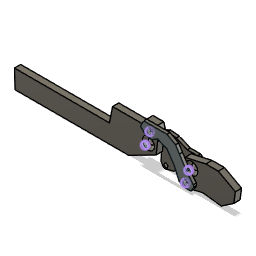
TestFingerJoint (Autodesk Fusion 360 design; units mm, degrees)
Autodesk Fusion 360 part; units mm, degrees
sketch "Sketch6" plane through (0, 0, 0) normal (0, 0, 1) x (1, 0, 0)
  line L0 (0, 0) -> (40, 0)
  line L1 (40, 0) -> (40, 20)
  line L2 (40, 20) -> (0, 20)
  line L3 (0, 20) -> (0, 0)
  line L4 (48, 20) -> (68, 20)
  line L5 (68, 20) -> (68, 0)
  line L6 (68, 0) -> (48, 0)
  line L7 (48, 0) -> (48, 20)
  line L8 (48, 13) -> (18, 13)
  line L9 (18, 13) -> (18, 7)
  line L10 (18, 7) -> (48, 7)
  line L11 (48, 7) -> (48, 13)
  line L12 (68, 13) -> (98, 13)
  line L13 (98, 13) -> (98, 7)
  line L14 (98, 7) -> (68, 7)
  line L15 (68, 7) -> (68, 13)
  line L16 (76, 0) -> (106, 0)
  line L17 (106, 0) -> (106, 20)
  line L18 (106, 20) -> (76, 20)
  line L19 (76, 20) -> (76, 0)
  dimension "d15" = 40
  dimension "d16" = 20
  dimension "d17" = 20
  dimension "d18" = 20
  dimension "d19" = 8
  dimension "d20" = 6
  dimension "d21" = 30
  dimension "d22" = 7
  dimension "d26" = 7
  dimension "d27" = 6
  dimension "d28" = 30
  dimension "d29" = 30
  dimension "d30" = 20
  dimension "d31" = 8
  constraint horizontal L0
  constraint vertical L1
  constraint horizontal L2
  constraint vertical L3
  constraint coincident L0.start L3.end
  constraint horizontal L4
  constraint vertical L5
  constraint horizontal L6
  constraint vertical L7
  constraint collinear L0 L6
  constraint horizontal L8
  constraint vertical L9
  constraint horizontal L10
  constraint vertical L11
  constraint coincident L7 L8.start
  constraint horizontal L12
  constraint vertical L13
  constraint horizontal L14
  constraint vertical L15
  constraint coincident L5 L12.start
  constraint horizontal L16
  constraint vertical L17
  constraint horizontal L18
  constraint vertical L19
  constraint collinear L0 L16
  measures "d15" distance of L0.start L0.end
  measures "d16" distance of L0.start L2.end
  measures "d17" distance of L5.end L6.end
  measures "d18" distance of L4.start L6.end
  measures "d19" distance of L1 L7
  measures "d20" distance of L8 L10
  measures "d21" distance of L8.start L8.end
  measures "d22" distance of L6 L10
  measures "d26" distance of L6 L14
  measures "d27" distance of L12.end L13.end
  measures "d28" distance of L12.start L12.end
  measures "d29" distance of L16.start L16.end
  measures "d30" distance of L16.start L18.end
  measures "d31" distance of L5 L19
extrude "Extrude6" add sketch "Sketch6" along normal blind 20 contours L0 L1 L2 L3 L8 L9 L10 | L1 L8 L9 L10 | L12 L13 L14 L19 | L12 L13 L14 L16 L17 L18 L19 makes body 1 at (13.3333, 0, 6.6667) makes body 2 at (96, 20, 6.6667)
extrude "Extrude7" add sketch "Sketch6" along normal blind 20 separate body contours L1 L8 L9 L10 | L1 L7 L8 L10 L11 | L4 L5 L6 L7 L11 L15 | L5 L12 L14 L15 L19 | L12 L13 L14 L19 makes body 3
sketch "Sketch7" plane through (0, 20, 0) normal (0, 1, 0) x (-1, 0, 0)
  line L0 (-68, 0) -> (-48, 0)
  line L1 (-48, 0) -> (-48, 20)
  line L2 (-48, 20) -> (-68, 20)
  line L3 (-68, 20) -> (-68, 0)
  line L4 (-98, 0) -> (-68, 0)
  line L5 (-68, 0) -> (-68, 20)
  line L6 (-68, 20) -> (-98, 20)
  line L7 (-98, 20) -> (-98, 0)
  line L8 (-48, 0) -> (-18, 0)
  line L9 (-18, 0) -> (-18, 20)
  line L10 (-18, 20) -> (-48, 20)
  line L11 (-48, 20) -> (-48, 0)
  line L12 (-98, 20) -> (-68, 20)
  line L13 (-68, 20) -> (-68, 15)
  line L14 (-68, 15) -> (-98, 15)
  line L15 (-98, 15) -> (-98, 20)
  line L16 (-98, 0) -> (-68, 0)
  line L17 (-68, 0) -> (-68, 5)
  line L18 (-68, 5) -> (-98, 5)
  line L19 (-98, 5) -> (-98, 0)
  line L20 (-48, 0) -> (-18, 0)
  line L21 (-18, 0) -> (-18, 5)
  line L22 (-18, 5) -> (-48, 5)
  line L23 (-48, 5) -> (-48, 0)
  line L24 (-18, 20) -> (-48, 20)
  line L25 (-48, 20) -> (-48, 15)
  line L26 (-48, 15) -> (-18, 15)
  line L27 (-18, 15) -> (-18, 20)
  dimension "d36" = 5
  dimension "d37" = 5
  dimension "d38" = 5
  dimension "d39" = 5
  constraint horizontal L12
  constraint vertical L13
  constraint horizontal L14
  constraint vertical L15
  constraint coincident L3 L13.end
  constraint coincident L6.end L7.start
  constraint horizontal L16
  constraint vertical L17
  constraint horizontal L18
  constraint vertical L19
  constraint coincident L5 L17.end
  constraint coincident L4.start L7.end
  constraint horizontal L20
  constraint vertical L21
  constraint horizontal L22
  constraint vertical L23
  constraint coincident L9 L21.end
  constraint coincident L0.end L1.start
  constraint horizontal L24
  constraint vertical L25
  constraint horizontal L26
  constraint vertical L27
  constraint coincident L11 L25.end
  constraint coincident L9.end L10.start
  measures "d36" distance of L6.end L14.end
  measures "d37" distance of L9.end L26.end
  measures "d38" distance of L4.start L18.end
  measures "d39" distance of L8.end L21.end
extrude "Extrude8" cut sketch "Sketch7" against normal blind 20 contours L3 L4 L5 L7 L16 L17 L18 L19 | L1 L8 L9 L11 L20 L21 L22 L23 | L3 L5 L6 L7 L12 L13 L14 L15 | L1 L9 L10 L11 L24 L25 L26 L27 bodies 3
sketch "Sketch8" plane through (0, 20, 0) normal (0, 1, 0) x (-1, 0, 0)
  line L0 (-40, 0) -> (0, 0)
  line L1 (0, 0) -> (0, 20)
  line L2 (0, 20) -> (-40, 20)
  line L3 (-40, 20) -> (-40, 0)
  line L4 (-103, 15.5) -> (-15, 15.5)
  line L5 (-15, 15.5) -> (-15, 4.5)
  line L6 (-15, 4.5) -> (-103, 4.5)
  line L7 (-103, 4.5) -> (-103, 15.5)
  line L8 (-98, 5) -> (-98, 15)
  line L9 (-68, 20) -> (-48, 20)
  point P0 (-18, 15)
  dimension "d43" = 5
  dimension "d44" = 3
  dimension "d45" = 11
  dimension "d46" = 4.5
  constraint horizontal L4
  constraint vertical L5
  constraint horizontal L6
  constraint vertical L7
  measures "d43" distance of L7 L8
  measures "d44" distance of L5 P0
  measures "d45" distance of L4.start L6.end
  measures "d46" distance of L4 L9
extrude "Extrude9" cut sketch "Sketch8" against normal blind 20 contours L3 L4 L6 L7 | L3 L4 L5 L6 bodies 1 2
sketch "Sketch9" plane through (0, 0, 20) normal (0, 0, 1) x (1, 0, 0)
  line L0 (0, 20) -> (0, 0)
  line L1 (0, 0) -> (40, 0)
  line L2 (40, 0) -> (40, 20)
  line L3 (40, 20) -> (0, 20)
  line L4 (98, 13) -> (68, 13)
  line L5 (68, 13) -> (68, 7)
  line L6 (68, 7) -> (98, 7)
  line L7 (98, 7) -> (98, 13)
  line L8 (48, 13) -> (18, 13)
  line L9 (18, 13) -> (18, 7)
  line L10 (18, 7) -> (48, 7)
  line L11 (48, 7) -> (48, 13)
  circle A0 centre (21.5, 10) radius 2
  circle A1 centre (94.5, 10) radius 2
  dimension "d49" = 4
  dimension "d50" = 4
  dimension "d51" = 3.5
  dimension "d52" = 3.5
  dimension "d53" = 3
  dimension "d54" = 3
  measures "d49" diameter of A0
  measures "d50" diameter of A1
  measures "d51" distance of L9 A0.centre
  measures "d52" distance of L7 A1.centre
  measures "d53" distance of L4 A1.centre
  measures "d54" distance of L10 A0.centre
extrude "Extrude10" cut sketch "Sketch9" against normal blind 20 contours A0 | A1 bodies 1 2 3
fillet "Fillet1" radius 8 8 edges at (40, 20, 2.25) (40, 20, 17.75) (40, 0, 17.75) (40, 0, 2.25) (76, 20, 17.75) (76, 20, 2.25) (76, 0, 17.75) (76, 0, 2.25) on bodies 1 2
fillet "Fillet2" radius 5 4 edges at (48, 0, 10) (68, 0, 10) (68, 20, 10) (48, 20, 10) on bodies 3
fillet "Fillet3" radius 4 4 edges at (48, 10, 15) (68, 10, 15) (68, 10, 5) (48, 10, 5) on bodies 3
sketch "Sketch10" plane through (0, 0, 20) normal (0, 0, 1) x (1, 0, 0)
  arc A0 (32, 0) -> (40, 8) centre (32, 8) ccw
  line L0 (40, 8) -> (40, 12)
  arc A1 (40, 12) -> (32, 20) centre (32, 12) ccw
  line L1 (32, 20) -> (0, 20)
  line L2 (0, 20) -> (0, 0)
  line L3 (0, 0) -> (32, 0)
  circle A2 centre (21.5, 10) radius 2
  line L4 (22.4525, 22.3546) -> (97.1627, 3.9644)
  line L5 (97.1627, 3.9644) -> (95.5692, -2.509)
  line L6 (95.5692, -2.509) -> (20.859, 15.8812)
  line L7 (20.859, 15.8812) -> (22.4525, 22.3546)
  line L8 (84, 0) -> (106, 0)
  circle A3 centre (94.5, 10) radius 2
  circle A4 centre (25.5, 18) radius 2
  circle A5 centre (90.5, 2) radius 2
  circle A6 centre (94.5, 10) radius 2
  dimension "d63" = 6.6667
  dimension "d66" = 4
  dimension "d67" = 4
  dimension "d96" = 8
  dimension "d98" = 8
  dimension "d99" = 4
  dimension "d100" = 6
  dimension "d101" = 3.5
  dimension "d103" = 4
  dimension "d104" = 3.5
  dimension "d105" = 4
  constraint perpendicular L4 L5
  constraint perpendicular L6 L7
  constraint perpendicular L5 L6
  measures "d63" distance of L4 L6
  measures "d66" diameter of A4
  measures "d67" diameter of A5
  measures "d96" vertical distance of A3.centre A5.centre
  measures "d98" vertical distance of A2.centre A4.centre
  measures "d99" distance of L7 A4.centre
  measures "d100" distance of L5 A5.centre
  measures "d101" distance of L4 A5.centre
  measures "d103" horizontal distance of A2.centre A4.centre
  measures "d104" distance of L4 A4.centre
  measures "d105" horizontal distance of A5.centre A3.centre
extrude "Extrude11" add sketch "Sketch10" along normal blind 3 separate body contours L0 A1 L1 L4 L6 L7 | L0 A1 L4 L5 L6 L8 | L5 L6 L8 | A1 L1 L4 L7 makes body 4
extrude "Extrude12" cut sketch "Sketch10" against normal blind 20 contours A4 | A5 bodies 1 2
chamfer "Chamfer1" distance 2 angle 45 2 edges at (19.6353, 10.7232, 20) (92.6353, 10.7232, 20) on bodies 1 2
fillet "Fillet4" radius 3 4 edges at (18, 13, 10) (98, 13, 10) (18, 7, 10) (98, 7, 10) on bodies 3
fillet "Fillet5" radius 2 4 edges at (20.859, 15.8812, 21.5) (22.4525, 22.3546, 21.5) (97.1627, 3.9644, 21.5) (95.5692, -2.509, 21.5) on bodies 4
copy_body "Body->Comp1" bodies 1 removing the originals makes body 5 in component "Component"
copy_body "Body->Comp2" bodies 2 removing the originals makes body 6 in component "Component'"
copy_body "Body->Comp3" bodies 3 removing the originals makes body 7 in component "Component''"
copy_body "Body->Comp4" bodies 4 removing the originals makes body 8 in component "Component'''"
sketch "Sketch11" plane through (0, 0, 0) normal (0, 0, 1) x (1, 0, 0)
  line L0 (7, 19) -> (7, -3)
  line L1 (7, -3) -> (17.4217, -3)
  line L2 (17.4217, -3) -> (35, 6)
  line L3 (35, 6) -> (36, 14)
  line L4 (27, 19) -> (7, 19)
  line L5 (67, 17) -> (53.6443, 14)
  line L6 (53.6443, 14) -> (50.5462, 8.5837)
  line L7 (50.5462, 8.5837) -> (52, -1)
  line L8 (65, 0) -> (76.9497, -1.4937)
  line L9 (76.9497, -1.4937) -> (85, 4)
  line L10 (85, 4) -> (86, 11)
  line L11 (86, 11) -> (75, 17)
  line L12 (75, 17) -> (67, 17)
  line L13 (27, 19) -> (29, 23)
  line L14 (29, 23) -> (36, 23)
  line L15 (36, 23) -> (37, 19)
  line L16 (37, 19) -> (36, 14)
  line L17 (52, -1) -> (58.4026, -1.6282)
  line L18 (58.4026, -1.6282) -> (65, 0)
  constraint vertical L0
  constraint perpendicular L0 L1
  constraint perpendicular L3 L8
  constraint horizontal L12
  constraint horizontal L4
  constraint parallel L4 L14
extrude "Extrude13" add sketch "Sketch11" along normal blind 2 separate body makes body 9 at (17.1406, 11.6667, 0) makes body 10 at (61.8814, 10.3333, 0)
sketch "Sketch12" plane through (0, 0, 2) normal (0, 0, 1) x (1, 0, 0)
  line L0 (27, 19) -> (7, 19)
  line L1 (7, 19) -> (7, -3)
  line L2 (7, -3) -> (17.4217, -3)
  line L3 (17.4217, -3) -> (35, 6)
  line L4 (35, 6) -> (36, 14)
  line L5 (36, 14) -> (37, 19)
  line L6 (37, 19) -> (36, 23)
  line L7 (36, 23) -> (29, 23)
  line L8 (29, 23) -> (27, 19)
  line L9 (29, 23) -> (27, 19)
  line L10 (27, 19) -> (30, 16)
  line L11 (30, 16) -> (34, 15)
  line L12 (34, 15) -> (38.0159, 17.5)
  line L13 (38.0159, 17.5) -> (40.2914, 16.25)
  line L14 (40.2914, 16.25) -> (44, 15)
  line L15 (44, 15) -> (46, 12)
  line L16 (46, 12) -> (48.6074, 8.089)
  line L17 (48.6074, 8.089) -> (50.6634, 3.4975)
  line L18 (50.6634, 3.4975) -> (51.8645, 0.8152)
  line L19 (51.8645, 0.8152) -> (55.0151, -0.9155)
  line L20 (55.0151, -0.9155) -> (59.4478, -0.9155)
  line L21 (59.4478, -0.9155) -> (61.1353, 2.1564)
  line L22 (61.1353, 2.1564) -> (60.2916, 7.1489)
  line L23 (60.2916, 7.1489) -> (57.2315, 12.0174)
  line L24 (57.2315, 12.0174) -> (52, 16)
  line L25 (52, 16) -> (49.5037, 19.9716)
  line L26 (49.5037, 19.9716) -> (44, 23)
  line L27 (44, 23) -> (38, 23)
  line L28 (38, 23) -> (29, 23)
  constraint coincident L7.end L8.start
  constraint coincident L0.start L8.end
  constraint parallel L15 L16
  constraint parallel L17 L18
  constraint parallel L13 L19
  constraint horizontal L20
  constraint perpendicular L19 L21
  constraint parallel L23 L25
  constraint horizontal L27
  constraint parallel L7 L28
extrude "Extrude14" add sketch "Sketch12" along normal blind 2 separate body contours L5 L6 L7 L8 L9 L10 L11 L12 L28 | L5 L6 L12 L13 L14 L15 L16 L17 L18 L19 L20 L21 L22 L23 L24 L25 L26 L27 L28 makes body 11
sketch "Sketch13" plane through (0, 0, 4) normal (0, 0, 1) x (1, 0, 0)
  line L0 (44, 23) -> (29, 23)
  line L1 (29, 23) -> (27, 19)
  line L2 (27, 19) -> (30, 16)
  line L3 (30, 16) -> (34, 15)
  line L4 (34, 15) -> (38.0159, 17.5)
  line L5 (38.0159, 17.5) -> (40.2914, 16.25)
  line L6 (40.2914, 16.25) -> (44, 15)
  line L7 (44, 15) -> (48.6074, 8.089)
  line L8 (48.6074, 8.089) -> (51.8645, 0.8152)
  line L9 (51.8645, 0.8152) -> (55.0151, -0.9155)
  line L10 (55.0151, -0.9155) -> (59.4478, -0.9155)
  line L11 (59.4478, -0.9155) -> (61.1353, 2.1564)
  line L12 (61.1353, 2.1564) -> (60.2916, 7.1489)
  line L13 (60.2916, 7.1489) -> (57.2315, 12.0174)
  line L14 (57.2315, 12.0174) -> (52, 16)
  line L15 (52, 16) -> (49.5037, 19.9716)
  line L16 (49.5037, 19.9716) -> (44, 23)
  line L17 (29, 14) -> (25, 12)
  line L18 (25, 12) -> (24.3664, 7.5642)
  line L19 (24.3664, 7.5642) -> (28, 6)
  line L20 (28, 6) -> (34, 6)
  line L21 (34, 6) -> (35, 4)
  line L22 (35, 4) -> (39, 0)
  line L23 (39, 0) -> (45, -3)
  line L24 (45, -3) -> (49, -1)
  line L25 (49, -1) -> (51.995, 4.4521)
  line L26 (51.995, 4.4521) -> (56.2929, 6.3766)
  line L27 (56.2929, 6.3766) -> (58.9406, 7.5623)
  line L28 (58.9406, 7.5623) -> (62.1557, 9.5831)
  line L29 (62.1557, 9.5831) -> (60.9516, 12.272)
  line L30 (60.9516, 12.272) -> (57.6168, 14.914)
  line L31 (57.6168, 14.914) -> (51, 14.914)
  line L32 (51, 14.914) -> (44, 18)
  line L33 (44, 18) -> (38.3016, 18.5595)
  line L34 (38.3016, 18.5595) -> (33.6565, 16.457)
  line L35 (33.6565, 16.457) -> (30.1314, 14.8614)
  line L36 (30.1314, 14.8614) -> (29, 14)
  constraint horizontal L20
  constraint perpendicular L17 L21
  constraint parallel L17 L24
  constraint perpendicular L9 L25
  constraint perpendicular L8 L26
  constraint perpendicular L8 L27
  constraint perpendicular L13 L28
  constraint perpendicular L27 L29
  constraint horizontal L31
  constraint parallel L34 L35
extrude "Extrude15" add sketch "Sketch13" along normal blind 2 separate body contours L13 L14 L28 L29 L30 L31 | L3 L4 L5 L6 L7 L8 L13 L14 L25 L26 L27 L28 L31 L32 L33 L34 L35 | L3 L4 L5 L6 L7 L8 L17 L18 L19 L20 L21 L22 L23 L24 L25 L35 L36 makes body 12
extrude "Extrude16" add 2 faces at (61.8814, 10.3333, 0) (17.1406, 11.6667, 0) along direction (0, 0, -1) blind 2 on bodies 9 10 bodies 10 9 11 12
sketch "Sketch14" plane through (0, 0, 6) normal (0, 0, 1) x (1, 0, 0)
  line L0 (30.1314, 14.8614) -> (29, 14)
  line L1 (29, 14) -> (25, 12)
  line L2 (25, 12) -> (24.3664, 7.5642)
  line L3 (24.3664, 7.5642) -> (28, 6)
  line L4 (28, 6) -> (34, 6)
  line L5 (34, 6) -> (35, 4)
  line L6 (35, 4) -> (39, 0)
  line L7 (39, 0) -> (45, -3)
  line L8 (45, -3) -> (49, -1)
  line L9 (49, -1) -> (51.995, 4.4521)
  line L10 (51.995, 4.4521) -> (58.9406, 7.5623)
  line L11 (58.9406, 7.5623) -> (62.1557, 9.5831)
  line L12 (62.1557, 9.5831) -> (60.9516, 12.272)
  line L13 (60.9516, 12.272) -> (57.6168, 14.914)
  line L14 (57.6168, 14.914) -> (51, 14.914)
  line L15 (51, 14.914) -> (44, 18)
  line L16 (44, 18) -> (38.3016, 18.5595)
  line L17 (38.3016, 18.5595) -> (30.1314, 14.8614)
  circle A0 centre (58, 10) radius 1.85
  circle A1 centre (56, 2) radius 1.85
  circle A2 centre (30, 10) radius 1.85
  circle A3 centre (33, 19) radius 1.85
  dimension "d114" = 3.7
  dimension "d115" = 3.7
  dimension "d116" = 3.7
  dimension "d117" = 3.7
  measures "d114" diameter of A0
  measures "d115" diameter of A1
  measures "d116" diameter of A2
  measures "d117" diameter of A3
extrude "Extrude17" cut sketch "Sketch14" against normal blind 8 contours A0 | A1 | A2 | A3 bodies 9 10 11 12
chamfer "Chamfer2" distance 2 angle 45 2 edges at (28.2752, 10.669, 2) (56.2752, 10.669, 2) on bodies 9 10
move_body "Move1" bodies 12 to x (1, 0, 0) y (0, 1, 0) z (0, 0, 1) at (0, 0, -8)
sketch "Sketch15" plane through (0, 0, 4) normal (0, 0, 1) x (1, 0, 0)
  arc A0 (57.3996, 11.7499) -> (59.3165, 8.7002) centre (58, 10) ccw
  line L0 (57.3996, 11.7499) -> (57.2315, 12.0174)
  line L1 (57.2315, 12.0174) -> (52, 16)
  line L2 (52, 16) -> (49.5037, 19.9716)
  line L3 (49.5037, 19.9716) -> (44, 23)
  line L4 (44, 23) -> (29, 23)
  line L5 (29, 23) -> (27, 19)
  line L6 (27, 19) -> (30, 16)
  line L7 (30, 16) -> (34, 15)
  line L8 (34, 15) -> (38.0159, 17.5)
  line L9 (38.0159, 17.5) -> (40.2914, 16.25)
  line L10 (40.2914, 16.25) -> (44, 15)
  line L11 (44, 15) -> (48.6074, 8.089)
  line L12 (48.6074, 8.089) -> (51.8645, 0.8152)
  line L13 (51.8645, 0.8152) -> (55.0151, -0.9155)
  line L14 (55.0151, -0.9155) -> (59.4478, -0.9155)
  line L15 (59.4478, -0.9155) -> (61.1353, 2.1564)
  line L16 (61.1353, 2.1564) -> (60.2916, 7.1489)
  line L17 (60.2916, 7.1489) -> (59.3165, 8.7002)
  circle A1 centre (56, 2) radius 1.85
  circle A2 centre (33, 19) radius 1.85
  line L18 (56.4337, 9.0155) -> (60.9319, 3.36)
  line L19 (56.6883, 8.6954) -> (52, 16)
  constraint midpoint A0 L18.start
  constraint coincident L16 L18.end
  constraint coincident A0 L19.start
  constraint coincident L18 L19.start
  constraint coincident L1.end L2.start
extrude "Extrude18" cut sketch "Sketch15" against normal blind 2 contours A0 L16 L17 L18 | A0 L0 L1 L19 bodies 11
chamfer "Chamfer3" distance 2 angle 45 2 edges at (31.2752, 18.331, -2) (54.2752, 1.331, -2) on bodies 9 10
sketch "Sketch16" plane through (0, 0, 2) normal (0, 0, 1) x (1, 0, 0)
  line L0 (27, 19) -> (7, 19)
  line L1 (7, 19) -> (7, -3)
  line L2 (7, -3) -> (17.4217, -3)
  line L3 (17.4217, -3) -> (35, 6)
  line L4 (35, 6) -> (36, 14)
  line L5 (36, 14) -> (37, 19)
  line L6 (37, 19) -> (36, 23)
  line L7 (36, 23) -> (29, 23)
  line L8 (29, 23) -> (27, 19)
  circle A0 centre (33, 19) radius 1.85
  circle A1 centre (30, 10) radius 3.85
  line L9 (7, -3) -> (-55.6859, -3)
  line L10 (-55.6859, -3) -> (-57.0823, 34.1911)
  line L11 (-57.0823, 34.1911) -> (0.0915, 30.8262)
  line L12 (0.0915, 30.8262) -> (7, 19)
  constraint coincident L1.end L2.start
  constraint perpendicular L1 L9
  constraint coincident L0.end L1.start
extrude "Extrude19" add sketch "Sketch16" against normal blind 4 contours L1 L9 L10 L11 L12 bodies 9
sketch "Sketch17" plane through (0, 0, 2) normal (0, 0, 1) x (1, 0, 0)
  line L0 (27, 19) -> (7, 19)
  line L1 (7, 19) -> (0.0915, 30.8262)
  line L2 (0.0915, 30.8262) -> (-57.0823, 34.1911)
  line L3 (-57.0823, 34.1911) -> (-55.6859, -3)
  line L4 (-55.6859, -3) -> (17.4217, -3)
  line L5 (17.4217, -3) -> (35, 6)
  line L6 (35, 6) -> (36, 14)
  line L7 (36, 14) -> (37, 19)
  line L8 (37, 19) -> (36, 23)
  line L9 (36, 23) -> (29, 23)
  line L10 (29, 23) -> (27, 19)
  circle A0 centre (33, 19) radius 1.85
  circle A1 centre (30, 10) radius 3.85
  line L11 (-56.1315, 8.8703) -> (5, 8.8703)
  line L12 (5, 8.8703) -> (7, 19)
  constraint coincident L3 L11.start
  constraint horizontal L11
  constraint coincident L0.end L1.start
extrude "Extrude20" cut sketch "Sketch17" against normal blind 4 contours L1 L2 L3 L11 L12 bodies 9
sketch "Sketch18" plane through (0, 0, 2) normal (0, 0, 1) x (1, 0, 0)
  circle A0 centre (30, 10) radius 3.85
  circle A1 centre (33, 19) radius 1.85
  line L0 (7, 19) -> (5, 8.8703)
  line L1 (5, 8.8703) -> (-56.1315, 8.8703)
  line L2 (-56.1315, 8.8703) -> (-55.6859, -3)
  line L3 (-55.6859, -3) -> (17.4217, -3)
  line L4 (17.4217, -3) -> (35, 6)
  line L5 (35, 6) -> (36, 14)
  line L6 (36, 14) -> (37, 19)
  line L7 (37, 19) -> (36, 23)
  line L8 (36, 23) -> (29, 23)
  line L9 (29, 23) -> (27, 19)
  line L10 (27, 19) -> (7, 19)
  line L11 (-56.1315, 8.8703) -> (-6.3246, 8.8703)
  line L12 (-6.3246, 8.8703) -> (-6.3246, 2.9351)
  line L13 (-6.3246, 2.9351) -> (-56.1315, 2.9351)
  line L14 (-56.1315, 2.9351) -> (-56.1315, 8.8703)
  constraint horizontal L11
  constraint vertical L12
  constraint horizontal L13
  constraint vertical L14
  constraint coincident L1.end L2.start
extrude "Extrude21" add sketch "Sketch18" along normal blind 4 contours L1 L2 L11 L12 L13 bodies 9
extrude "Extrude22" add 1 faces at (-39.4549, 6.8919, 6) along direction (0, 0, 1) blind 4 on bodies 9 bodies 9
sketch "Sketch19" plane through (0, 0, -4) normal (0, 0, -1) x (-1, 0, 0)
  circle A0 centre (-30, 10) radius 1.85
  circle A1 centre (-58, 10) radius 1.85
  line L0 (-29, 14) -> (-30.1314, 14.8614)
  line L1 (-30.1314, 14.8614) -> (-38.3016, 18.5595)
  line L2 (-38.3016, 18.5595) -> (-44, 18)
  line L3 (-44, 18) -> (-51, 14.914)
  line L4 (-51, 14.914) -> (-57.6168, 14.914)
  line L5 (-57.6168, 14.914) -> (-60.9516, 12.272)
  line L6 (-60.9516, 12.272) -> (-62.1557, 9.5831)
  line L7 (-62.1557, 9.5831) -> (-58.9406, 7.5623)
  line L8 (-58.9406, 7.5623) -> (-51.995, 4.4521)
  line L9 (-51.995, 4.4521) -> (-49, -1)
  line L10 (-49, -1) -> (-45, -3)
  line L11 (-45, -3) -> (-39, 0)
  line L12 (-39, 0) -> (-35, 4)
  line L13 (-35, 4) -> (-34, 6)
  line L14 (-34, 6) -> (-28, 6)
  line L15 (-28, 6) -> (-24.3664, 7.5642)
  line L16 (-24.3664, 7.5642) -> (-25, 12)
  line L17 (-25, 12) -> (-29, 14)
  line L18 (-51.995, 4.4521) -> (-42, -1.5)
  constraint coincident L8.end L9.start
  constraint midpoint L11 L18.end
extrude "Extrude23" cut sketch "Sketch19" against normal blind 2 contours L9 L10 L11 L18 bodies 12
sketch "Sketch20" plane through (0, 0, -4) normal (0, 0, -1) x (-1, 0, 0)
  line L0 (-51.995, 4.4521) -> (-42, -1.5)
  line L1 (-42, -1.5) -> (-39, 0)
  line L2 (-39, 0) -> (-35, 4)
  line L3 (-35, 4) -> (-34, 6)
  line L4 (-34, 6) -> (-28, 6)
  line L5 (-28, 6) -> (-24.3664, 7.5642)
  line L6 (-24.3664, 7.5642) -> (-25, 12)
  line L7 (-25, 12) -> (-29, 14)
  line L8 (-29, 14) -> (-30.1314, 14.8614)
  line L9 (-30.1314, 14.8614) -> (-38.3016, 18.5595)
  line L10 (-38.3016, 18.5595) -> (-44, 18)
  line L11 (-44, 18) -> (-51, 14.914)
  line L12 (-51, 14.914) -> (-57.6168, 14.914)
  line L13 (-57.6168, 14.914) -> (-60.9516, 12.272)
  line L14 (-60.9516, 12.272) -> (-62.1557, 9.5831)
  line L15 (-62.1557, 9.5831) -> (-58.9406, 7.5623)
  line L16 (-58.9406, 7.5623) -> (-51.995, 4.4521)
  circle A0 centre (-30, 10) radius 1.85
  circle A1 centre (-58, 10) radius 1.85
  line L17 (-42, -1.5) -> (-36, -3)
  line L18 (-36, -3) -> (-34.141, 0.1217)
  line L19 (-34.141, 0.1217) -> (-34.5, 5)
  constraint coincident L0.end L1.start
  constraint perpendicular L0 L18
  constraint midpoint L3 L19.end
extrude "Extrude24" add sketch "Sketch20" against normal blind 2 contours L1 L2 L3 L17 L18 L19 bodies 12
sketch "Sketch21" plane through (0, 0, -4) normal (0, 0, -1) x (-1, 0, 0)
  line L0 (-51.995, 4.4521) -> (-42, -1.5)
  line L1 (-42, -1.5) -> (-36, -3)
  line L2 (-36, -3) -> (-34.141, 0.1217)
  line L3 (-34.141, 0.1217) -> (-34.5, 5)
  line L4 (-34.5, 5) -> (-34, 6)
  line L5 (-34, 6) -> (-28, 6)
  line L6 (-28, 6) -> (-24.3664, 7.5642)
  line L7 (-24.3664, 7.5642) -> (-25, 12)
  line L8 (-25, 12) -> (-29, 14)
  line L9 (-29, 14) -> (-30.1314, 14.8614)
  line L10 (-30.1314, 14.8614) -> (-38.3016, 18.5595)
  line L11 (-38.3016, 18.5595) -> (-44, 18)
  line L12 (-44, 18) -> (-51, 14.914)
  line L13 (-51, 14.914) -> (-57.6168, 14.914)
  line L14 (-57.6168, 14.914) -> (-60.9516, 12.272)
  line L15 (-60.9516, 12.272) -> (-62.1557, 9.5831)
  line L16 (-62.1557, 9.5831) -> (-58.9406, 7.5623)
  line L17 (-58.9406, 7.5623) -> (-51.995, 4.4521)
  circle A0 centre (-30, 10) radius 1.85
  circle A1 centre (-58, 10) radius 1.85
  circle A2 centre (-37.3245, -0.6644) radius 1.25
  dimension "d136" = 2.5
  measures "d136" diameter of A2
extrude "Extrude25" cut sketch "Sketch21" against normal blind 2 contours A2 bodies 12
fillet "Fillet6" radius 1 1 edges at (36, -3, -3) on bodies 12
extrude "Extrude26" cut 1 faces at (-39.4549, 6.8919, 10) along direction (0, 0, -1) blind 8 on bodies 9 bodies 9
copy_body "Body->Comp5" bodies 9 removing the originals makes body 13 in component "Component''''"
copy_body "Body->Comp6" bodies 10 removing the originals makes body 14 in component "Component'''''"
copy_body "Body->Comp7" bodies 11 removing the originals makes body 15 in component "Component''''''"
copy_body "Body->Comp8" bodies 12 removing the originals makes body 16 in component "Component'''''''"
sketch "Sketch22" plane through (0, 0, 4) normal (0, 0, 1) x (1, 0, 0)
  line L0 (56.2677, 9.3508) -> (52, 16)
  line L1 (52, 16) -> (49.5037, 19.9716)
  line L2 (49.5037, 19.9716) -> (44, 23)
  line L3 (44, 23) -> (29, 23)
  line L4 (29, 23) -> (27, 19)
  line L5 (27, 19) -> (30, 16)
  line L6 (30, 16) -> (34, 15)
  line L7 (34, 15) -> (38.0159, 17.5)
  line L8 (38.0159, 17.5) -> (40.2914, 16.25)
  line L9 (40.2914, 16.25) -> (44, 15)
  line L10 (44, 15) -> (48.6074, 8.089)
  line L11 (48.6074, 8.089) -> (51.8645, 0.8152)
  line L12 (51.8645, 0.8152) -> (55.0151, -0.9155)
  line L13 (55.0151, -0.9155) -> (59.4478, -0.9155)
  line L14 (59.4478, -0.9155) -> (61.1353, 2.1564)
  line L15 (61.1353, 2.1564) -> (60.9319, 3.36)
  line L16 (60.9319, 3.36) -> (56.6883, 8.6954)
  arc A0 (56.2677, 9.3508) -> (56.6883, 8.6954) centre (58, 10) ccw
  circle A1 centre (56, 2) radius 1.85
  circle A2 centre (33, 19) radius 1.85
  circle A3 centre (33, 19) radius 1.85
  circle A4 centre (30, 10) radius 1.85
  circle A5 centre (58, 10) radius 1.85
  circle A6 centre (56, 2) radius 1.85
  dimension "d159" = 9
  dimension "d160" = 8
  dimension "d161" = 3
  dimension "d162" = 2
  measures "d159" vertical distance of A2.centre A4.centre
  measures "d160" vertical distance of A0.centre A1.centre
  measures "d161" horizontal distance of A2.centre A4.centre
  measures "d162" horizontal distance of A1.centre A0.centre
component "Component" placed x (1, 0, 0) y (0, 1, 0) z (0, 0, 1) at (0, 0, 0)
component "Component'" placed x (1, 0, 0) y (0, 1, 0) z (0, 0, 1) at (0, 0, 0)
component "Component''" placed x (1, 0, 0) y (0, 1, 0) z (0, 0, 1) at (0, 0, 0)
component "Component'''" placed x (1, 0, 0) y (0, 1, 0) z (0, 0, 1) at (0, 0, 0)
component "Component''''" placed x (1, 0, 0) y (0, 1, 0) z (0, 0, 1) at (0, 0, 0)
component "Component'''''" placed x (1, 0, 0) y (0, 1, 0) z (0, 0, 1) at (0, 0, 0)
component "Component''''''" placed x (1, 0, 0) y (0, 1, 0) z (0, 0, 1) at (0, 0, 0)
component "Component'''''''" placed x (1, 0, 0) y (0, 1, 0) z (0, 0, 1) at (0, 0, 0)
equation "d15 = first_joint_length"
equation "d16 = finger_thickness"
equation "d17 = first_joint_length / 4 * 2"
equation "d18 = finger_thickness"
equation "d20 = joint_thickness"
equation "d22 = ( finger_thickness - joint_thickness ) / 2"
equation "first_joint_length = 40 mm"
equation "finger_thickness = 20 mm"
equation "joint_thickness = 6 mm"
equation "d26 = d22"
equation "d27 = d20"
equation "d28 = d21"
equation "d29 = d15 / 4 * 3"
equation "d30 = d18"
equation "d31 = d19"
equation "d32 = finger_thickness"
equation "d36 = d37"
equation "d37 = finger_thickness / 4"
equation "d38 = d37"
equation "d39 = d37"
equation "d45 = finger_thickness / 2 + 1 mm"
equation "d46 = finger_thickness / 4 - 0.5 mm"
equation "d63 = finger_thickness / 3"
